Autodesk Fusion 360 part; units mm, degrees
(part 18 of 18)
  line L11330 (212.0954, -1.666) -> (212.0954, -1.906)
  line L11331 (211.6754, -1.666) -> (212.0954, -1.666)
  line L11332 (211.6754, -2.1661) -> (212.0954, -2.1661)
  line L11333 (212.0954, -2.1661) -> (212.0954, -2.4061)
  line L11334 (212.0954, -2.4061) -> (211.6754, -2.4061)
  line L11335 (211.6754, -2.4061) -> (211.6754, -2.1661)
  line L11336 (212.0954, -2.906) -> (211.6754, -2.906)
  line L11337 (211.6754, -2.666) -> (212.0954, -2.666)
  line L11338 (211.6754, -2.906) -> (211.6754, -2.666)
  line L11339 (212.0954, -2.666) -> (212.0954, -2.906)
  line L11340 (212.0954, -3.4059) -> (211.6754, -3.4059)
  line L11341 (211.6754, -3.1659) -> (212.0954, -3.1659)
  line L11342 (212.0954, -3.1659) -> (212.0954, -3.4059)
  line L11343 (211.6754, -3.4059) -> (211.6754, -3.1659)
  line L11344 (138.9953, -77.1606) -> (138.9953, -76.5606)
  line L11345 (138.7753, -77.1606) -> (138.9953, -77.1606)
  line L11346 (138.7753, -76.5606) -> (138.7753, -77.1606)
  line L11347 (138.9953, -76.5606) -> (138.7753, -76.5606)
  line L11348 (141.8953, -76.5606) -> (141.8953, -77.1606)
  line L11349 (141.6753, -77.1606) -> (141.6753, -76.5606)
  line L11350 (141.8953, -77.1606) -> (141.6753, -77.1606)
  line L11351 (141.6753, -76.5606) -> (141.8953, -76.5606)
  line L11352 (138.9953, -19.985) -> (138.9953, -19.385)
  line L11353 (138.7753, -19.385) -> (138.7753, -19.985)
  line L11354 (138.7753, -19.985) -> (138.9953, -19.985)
  line L11355 (138.9953, -19.385) -> (138.7753, -19.385)
  line L11356 (141.6753, -19.985) -> (141.6753, -19.385)
  line L11357 (141.8953, -19.985) -> (141.6753, -19.985)
  line L11358 (141.8953, -19.385) -> (141.8953, -19.985)
  line L11359 (141.6753, -19.385) -> (141.8953, -19.385)
  line L11360 (138.9953, -39.0351) -> (138.9953, -38.4351)
  line L11361 (138.7753, -39.0351) -> (138.9953, -39.0351)
  line L11362 (138.7753, -38.4351) -> (138.7753, -39.0351)
  line L11363 (138.9953, -38.4351) -> (138.7753, -38.4351)
  line L11364 (141.6753, -38.4351) -> (141.8953, -38.4351)
  line L11365 (141.6753, -39.0351) -> (141.6753, -38.4351)
  line L11366 (141.8953, -39.0351) -> (141.6753, -39.0351)
  line L11367 (141.8953, -38.4351) -> (141.8953, -39.0351)
  line L11368 (138.7753, -58.0978) -> (138.9953, -58.0978)
  line L11369 (138.9953, -58.0978) -> (138.9953, -57.4978)
  line L11370 (138.9953, -57.4978) -> (138.7753, -57.4978)
  line L11371 (138.7753, -57.4978) -> (138.7753, -58.0978)
  line L11372 (141.6753, -57.4978) -> (141.8953, -57.4978)
  line L11373 (141.8953, -57.4978) -> (141.8953, -58.0978)
  line L11374 (141.6753, -58.0978) -> (141.6753, -57.4978)
  line L11375 (141.8953, -58.0978) -> (141.6753, -58.0978)
  line L11376 (157.8253, -19.385) -> (157.8253, -19.985)
  line L11377 (157.8253, -19.985) -> (158.0453, -19.985)
  line L11378 (158.0453, -19.385) -> (157.8253, -19.385)
  line L11379 (158.0453, -19.985) -> (158.0453, -19.385)
  line L11380 (160.9453, -19.985) -> (160.7253, -19.985)
  line L11381 (160.7253, -19.985) -> (160.7253, -19.385)
  line L11382 (160.9453, -19.385) -> (160.9453, -19.985)
  line L11383 (160.7253, -19.385) -> (160.9453, -19.385)
  line L11384 (158.0453, -76.5606) -> (157.8253, -76.5606)
  line L11385 (157.8253, -77.1606) -> (158.0453, -77.1606)
  line L11386 (158.0453, -77.1606) -> (158.0453, -76.5606)
  line L11387 (157.8253, -76.5606) -> (157.8253, -77.1606)
  line L11388 (160.9453, -76.5606) -> (160.9453, -77.1606)
  line L11389 (160.9453, -77.1606) -> (160.7253, -77.1606)
  line L11390 (160.7253, -77.1606) -> (160.7253, -76.5606)
  line L11391 (160.7253, -76.5606) -> (160.9453, -76.5606)
  line L11392 (157.8253, -57.4978) -> (157.8253, -58.0978)
  line L11393 (157.8253, -58.0978) -> (158.0453, -58.0978)
  line L11394 (158.0453, -57.4978) -> (157.8253, -57.4978)
  line L11395 (158.0453, -58.0978) -> (158.0453, -57.4978)
  line L11396 (160.7253, -58.0978) -> (160.7253, -57.4978)
  line L11397 (160.9453, -58.0978) -> (160.7253, -58.0978)
  line L11398 (160.7253, -57.4978) -> (160.9453, -57.4978)
  line L11399 (160.9453, -57.4978) -> (160.9453, -58.0978)
  line L11400 (158.0453, -38.4351) -> (157.8253, -38.4351)
  line L11401 (157.8253, -38.4351) -> (157.8253, -39.0351)
  line L11402 (158.0453, -39.0351) -> (158.0453, -38.4351)
  line L11403 (157.8253, -39.0351) -> (158.0453, -39.0351)
  line L11404 (160.7253, -38.4351) -> (160.9453, -38.4351)
  line L11405 (160.7253, -39.0351) -> (160.7253, -38.4351)
  line L11406 (160.9453, -38.4351) -> (160.9453, -39.0351)
  line L11407 (160.9453, -39.0351) -> (160.7253, -39.0351)
  line L11408 (177.0954, -19.385) -> (176.8754, -19.385)
  line L11409 (176.8754, -19.385) -> (176.8754, -19.985)
  line L11410 (177.0954, -19.985) -> (177.0954, -19.385)
  line L11411 (176.8754, -19.985) -> (177.0954, -19.985)
  line L11412 (179.7754, -19.385) -> (179.9954, -19.385)
  line L11413 (179.7754, -19.985) -> (179.7754, -19.385)
  line L11414 (179.9954, -19.985) -> (179.7754, -19.985)
  line L11415 (179.9954, -19.385) -> (179.9954, -19.985)
  line L11416 (177.0954, -76.5606) -> (176.8754, -76.5606)
  line L11417 (176.8754, -77.1606) -> (177.0954, -77.1606)
  line L11418 (177.0954, -77.1606) -> (177.0954, -76.5606)
  line L11419 (176.8754, -76.5606) -> (176.8754, -77.1606)
  line L11420 (179.7754, -76.5606) -> (179.9954, -76.5606)
  line L11421 (179.9954, -77.1606) -> (179.7754, -77.1606)
  line L11422 (179.9954, -76.5606) -> (179.9954, -77.1606)
  line L11423 (179.7754, -77.1606) -> (179.7754, -76.5606)
  line L11424 (177.0954, -58.0978) -> (177.0954, -57.4978)
  line L11425 (176.8754, -57.4978) -> (176.8754, -58.0978)
  line L11426 (176.8754, -58.0978) -> (177.0954, -58.0978)
  line L11427 (177.0954, -57.4978) -> (176.8754, -57.4978)
  line L11428 (179.9954, -57.4978) -> (179.9954, -58.0978)
  line L11429 (179.9954, -58.0978) -> (179.7754, -58.0978)
  line L11430 (179.7754, -58.0978) -> (179.7754, -57.4978)
  line L11431 (179.7754, -57.4978) -> (179.9954, -57.4978)
  line L11432 (176.8754, -38.4351) -> (176.8754, -39.0351)
  line L11433 (177.0954, -38.4351) -> (176.8754, -38.4351)
  line L11434 (177.0954, -39.0351) -> (177.0954, -38.4351)
  line L11435 (176.8754, -39.0351) -> (177.0954, -39.0351)
  line L11436 (179.9954, -38.4351) -> (179.9954, -39.0351)
  line L11437 (179.7754, -39.0351) -> (179.7754, -38.4351)
  line L11438 (179.7754, -38.4351) -> (179.9954, -38.4351)
  line L11439 (179.9954, -39.0351) -> (179.7754, -39.0351)
  line L11440 (100.8952, -77.1606) -> (100.8952, -76.5606)
  line L11441 (100.6752, -76.5606) -> (100.6752, -77.1606)
  line L11442 (100.6752, -77.1606) -> (100.8952, -77.1606)
  line L11443 (100.8952, -76.5606) -> (100.6752, -76.5606)
  line L11444 (103.7952, -77.1606) -> (103.5752, -77.1606)
  line L11445 (103.7952, -76.5606) -> (103.7952, -77.1606)
  line L11446 (103.5752, -77.1606) -> (103.5752, -76.5606)
  line L11447 (103.5752, -76.5606) -> (103.7952, -76.5606)
  line L11448 (100.6752, -58.0978) -> (100.8952, -58.0978)
  line L11449 (100.8952, -57.4978) -> (100.6752, -57.4978)
  line L11450 (100.8952, -58.0978) -> (100.8952, -57.4978)
  line L11451 (100.6752, -57.4978) -> (100.6752, -58.0978)
  line L11452 (103.5752, -58.0978) -> (103.5752, -57.4978)
  line L11453 (103.7952, -57.4978) -> (103.7952, -58.0978)
  line L11454 (103.7952, -58.0978) -> (103.5752, -58.0978)
  line L11455 (103.5752, -57.4978) -> (103.7952, -57.4978)
  line L11456 (100.8952, -19.985) -> (100.8952, -19.385)
  line L11457 (100.8952, -19.385) -> (100.6752, -19.385)
  line L11458 (100.6752, -19.985) -> (100.8952, -19.985)
  line L11459 (100.6752, -19.385) -> (100.6752, -19.985)
  line L11460 (103.5752, -19.385) -> (103.7952, -19.385)
  line L11461 (103.7952, -19.985) -> (103.5752, -19.985)
  line L11462 (103.7952, -19.385) -> (103.7952, -19.985)
  line L11463 (103.5752, -19.985) -> (103.5752, -19.385)
  line L11464 (100.6752, -39.0351) -> (100.8952, -39.0351)
  line L11465 (100.8952, -39.0351) -> (100.8952, -38.4351)
  line L11466 (100.8952, -38.4351) -> (100.6752, -38.4351)
  line L11467 (100.6752, -38.4351) -> (100.6752, -39.0351)
  line L11468 (103.5752, -39.0351) -> (103.5752, -38.4351)
  line L11469 (103.5752, -38.4351) -> (103.7952, -38.4351)
  line L11470 (103.7952, -38.4351) -> (103.7952, -39.0351)
  line L11471 (103.7952, -39.0351) -> (103.5752, -39.0351)
  line L11472 (119.7252, -19.385) -> (119.7252, -19.985)
  line L11473 (119.9452, -19.985) -> (119.9452, -19.385)
  line L11474 (119.9452, -19.385) -> (119.7252, -19.385)
  line L11475 (119.7252, -19.985) -> (119.9452, -19.985)
  line L11476 (122.6252, -19.385) -> (122.8452, -19.385)
  line L11477 (122.6252, -19.985) -> (122.6252, -19.385)
  line L11478 (122.8452, -19.385) -> (122.8452, -19.985)
  line L11479 (122.8452, -19.985) -> (122.6252, -19.985)
  line L11480 (119.7252, -57.4978) -> (119.7252, -58.0978)
  line L11481 (119.9452, -57.4978) -> (119.7252, -57.4978)
  line L11482 (119.9452, -58.0978) -> (119.9452, -57.4978)
  line L11483 (119.7252, -58.0978) -> (119.9452, -58.0978)
  line L11484 (122.6252, -57.4978) -> (122.8452, -57.4978)
  line L11485 (122.6252, -58.0978) -> (122.6252, -57.4978)
  line L11486 (122.8452, -57.4978) -> (122.8452, -58.0978)
  line L11487 (122.8452, -58.0978) -> (122.6252, -58.0978)
  line L11488 (119.9452, -39.0351) -> (119.9452, -38.4351)
  line L11489 (119.9452, -38.4351) -> (119.7252, -38.4351)
  line L11490 (119.7252, -38.4351) -> (119.7252, -39.0351)
  line L11491 (119.7252, -39.0351) -> (119.9452, -39.0351)
  line L11492 (122.8452, -38.4351) -> (122.8452, -39.0351)
  line L11493 (122.8452, -39.0351) -> (122.6252, -39.0351)
  line L11494 (122.6252, -38.4351) -> (122.8452, -38.4351)
  line L11495 (122.6252, -39.0351) -> (122.6252, -38.4351)
  line L11496 (119.9452, -76.5606) -> (119.7252, -76.5606)
  line L11497 (119.9452, -77.1606) -> (119.9452, -76.5606)
  line L11498 (119.7252, -77.1606) -> (119.9452, -77.1606)
  line L11499 (119.7252, -76.5606) -> (119.7252, -77.1606)
  line L11500 (122.6252, -76.5606) -> (122.8452, -76.5606)
  line L11501 (122.6252, -77.1606) -> (122.6252, -76.5606)
  line L11502 (122.8452, -76.5606) -> (122.8452, -77.1606)
  line L11503 (122.8452, -77.1606) -> (122.6252, -77.1606)
  line L11504 (5.425, -76.5606) -> (5.425, -77.1606)
  line L11505 (5.425, -77.1606) -> (5.645, -77.1606)
  line L11506 (5.645, -76.5606) -> (5.425, -76.5606)
  line L11507 (5.645, -77.1606) -> (5.645, -76.5606)
  line L11508 (8.545, -76.5606) -> (8.545, -77.1606)
  line L11509 (8.325, -77.1606) -> (8.325, -76.5606)
  line L11510 (8.545, -77.1606) -> (8.325, -77.1606)
  line L11511 (8.325, -76.5606) -> (8.545, -76.5606)
  line L11512 (24.4751, -77.1606) -> (24.6951, -77.1606)
  line L11513 (24.4751, -76.5606) -> (24.4751, -77.1606)
  line L11514 (24.6951, -77.1606) -> (24.6951, -76.5606)
  line L11515 (24.6951, -76.5606) -> (24.4751, -76.5606)
  line L11516 (27.5951, -77.1606) -> (27.3751, -77.1606)
  line L11517 (27.3751, -76.5606) -> (27.5951, -76.5606)
  line L11518 (27.3751, -77.1606) -> (27.3751, -76.5606)
  line L11519 (27.5951, -76.5606) -> (27.5951, -77.1606)
  line L11520 (43.7451, -76.5606) -> (43.5251, -76.5606)
  line L11521 (43.5251, -76.5606) -> (43.5251, -77.1606)
  line L11522 (43.5251, -77.1606) -> (43.7451, -77.1606)
  line L11523 (43.7451, -77.1606) -> (43.7451, -76.5606)
  line L11524 (46.6451, -77.1606) -> (46.4251, -77.1606)
  line L11525 (46.6451, -76.5606) -> (46.6451, -77.1606)
  line L11526 (46.4251, -77.1606) -> (46.4251, -76.5606)
  line L11527 (46.4251, -76.5606) -> (46.6451, -76.5606)
  line L11528 (62.5751, -19.985) -> (62.7951, -19.985)
  line L11529 (62.5751, -19.385) -> (62.5751, -19.985)
  line L11530 (62.7951, -19.385) -> (62.5751, -19.385)
  line L11531 (62.7951, -19.985) -> (62.7951, -19.385)
  line L11532 (65.6951, -19.985) -> (65.4751, -19.985)
  line L11533 (65.4751, -19.985) -> (65.4751, -19.385)
  line L11534 (65.6951, -19.385) -> (65.6951, -19.985)
  line L11535 (65.4751, -19.385) -> (65.6951, -19.385)
  line L11536 (62.5751, -77.1606) -> (62.7951, -77.1606)
  line L11537 (62.5751, -76.5606) -> (62.5751, -77.1606)
  line L11538 (62.7951, -76.5606) -> (62.5751, -76.5606)
  line L11539 (62.7951, -77.1606) -> (62.7951, -76.5606)
  line L11540 (65.6951, -77.1606) -> (65.4751, -77.1606)
  line L11541 (65.6951, -76.5606) -> (65.6951, -77.1606)
  line L11542 (65.4751, -77.1606) -> (65.4751, -76.5606)
  line L11543 (65.4751, -76.5606) -> (65.6951, -76.5606)
  line L11544 (62.7951, -39.0351) -> (62.7951, -38.4351)
  line L11545 (62.7951, -38.4351) -> (62.5751, -38.4351)
  line L11546 (62.5751, -39.0351) -> (62.7951, -39.0351)
  line L11547 (62.5751, -38.4351) -> (62.5751, -39.0351)
  line L11548 (65.6951, -39.0351) -> (65.4751, -39.0351)
  line L11549 (65.6951, -38.4351) -> (65.6951, -39.0351)
  line L11550 (65.4751, -39.0351) -> (65.4751, -38.4351)
  line L11551 (65.4751, -38.4351) -> (65.6951, -38.4351)
  line L11552 (62.7951, -57.4978) -> (62.5751, -57.4978)
  line L11553 (62.7951, -58.0978) -> (62.7951, -57.4978)
  line L11554 (62.5751, -57.4978) -> (62.5751, -58.0978)
  line L11555 (62.5751, -58.0978) -> (62.7951, -58.0978)
  line L11556 (65.4751, -57.4978) -> (65.6951, -57.4978)
  line L11557 (65.6951, -57.4978) -> (65.6951, -58.0978)
  line L11558 (65.6951, -58.0978) -> (65.4751, -58.0978)
  line L11559 (65.4751, -58.0978) -> (65.4751, -57.4978)
  line L11560 (81.8452, -39.0351) -> (81.8452, -38.4351)
  line L11561 (81.6252, -38.4351) -> (81.6252, -39.0351)
  line L11562 (81.8452, -38.4351) -> (81.6252, -38.4351)
  line L11563 (81.6252, -39.0351) -> (81.8452, -39.0351)
  line L11564 (84.5252, -39.0351) -> (84.5252, -38.4351)
  line L11565 (84.7452, -38.4351) -> (84.7452, -39.0351)
  line L11566 (84.7452, -39.0351) -> (84.5252, -39.0351)
  line L11567 (84.5252, -38.4351) -> (84.7452, -38.4351)
  line L11568 (81.6252, -76.5606) -> (81.6252, -77.1606)
  line L11569 (81.6252, -77.1606) -> (81.8452, -77.1606)
  line L11570 (81.8452, -77.1606) -> (81.8452, -76.5606)
  line L11571 (81.8452, -76.5606) -> (81.6252, -76.5606)
  line L11572 (84.7452, -76.5606) -> (84.7452, -77.1606)
  line L11573 (84.7452, -77.1606) -> (84.5252, -77.1606)
  line L11574 (84.5252, -77.1606) -> (84.5252, -76.5606)
  line L11575 (84.5252, -76.5606) -> (84.7452, -76.5606)
  line L11576 (81.6252, -19.385) -> (81.6252, -19.985)
  line L11577 (81.8452, -19.985) -> (81.8452, -19.385)
  line L11578 (81.8452, -19.385) -> (81.6252, -19.385)
  line L11579 (81.6252, -19.985) -> (81.8452, -19.985)
  line L11580 (84.7452, -19.385) -> (84.7452, -19.985)
  line L11581 (84.7452, -19.985) -> (84.5252, -19.985)
  line L11582 (84.5252, -19.985) -> (84.5252, -19.385)
  line L11583 (84.5252, -19.385) -> (84.7452, -19.385)
  line L11584 (81.8452, -58.0978) -> (81.8452, -57.4978)
  line L11585 (81.6252, -57.4978) -> (81.6252, -58.0978)
  line L11586 (81.8452, -57.4978) -> (81.6252, -57.4978)
  line L11587 (81.6252, -58.0978) -> (81.8452, -58.0978)
  line L11588 (84.7452, -58.0978) -> (84.5252, -58.0978)
  line L11589 (84.7452, -57.4978) -> (84.7452, -58.0978)
  line L11590 (84.5252, -57.4978) -> (84.7452, -57.4978)
  line L11591 (84.5252, -58.0978) -> (84.5252, -57.4978)
  line L11592 (5.425, -57.4978) -> (5.425, -58.0978)
  line L11593 (5.645, -58.0978) -> (5.645, -57.4978)
  line L11594 (5.425, -58.0978) -> (5.645, -58.0978)
  line L11595 (5.645, -57.4978) -> (5.425, -57.4978)
  line L11596 (8.545, -57.4978) -> (8.545, -58.0978)
  line L11597 (8.545, -58.0978) -> (8.325, -58.0978)
  line L11598 (8.325, -57.4978) -> (8.545, -57.4978)
  line L11599 (8.325, -58.0978) -> (8.325, -57.4978)
  line L11600 (5.425, -19.985) -> (5.645, -19.985)
  line L11601 (5.425, -19.385) -> (5.425, -19.985)
  line L11602 (5.645, -19.385) -> (5.425, -19.385)
  line L11603 (5.645, -19.985) -> (5.645, -19.385)
  line L11604 (8.325, -19.985) -> (8.325, -19.385)
  line L11605 (8.545, -19.385) -> (8.545, -19.985)
  line L11606 (8.545, -19.985) -> (8.325, -19.985)
  line L11607 (8.325, -19.385) -> (8.545, -19.385)
  line L11608 (5.425, -38.4351) -> (5.425, -39.0351)
  line L11609 (5.425, -39.0351) -> (5.645, -39.0351)
  line L11610 (5.645, -39.0351) -> (5.645, -38.4351)
  line L11611 (5.645, -38.4351) -> (5.425, -38.4351)
  line L11612 (8.325, -38.4351) -> (8.545, -38.4351)
  line L11613 (8.325, -39.0351) -> (8.325, -38.4351)
  line L11614 (8.545, -38.4351) -> (8.545, -39.0351)
  line L11615 (8.545, -39.0351) -> (8.325, -39.0351)
  line L11616 (24.6951, -38.4351) -> (24.4751, -38.4351)
  line L11617 (24.4751, -38.4351) -> (24.4751, -39.0351)
  line L11618 (24.4751, -39.0351) -> (24.6951, -39.0351)
  line L11619 (24.6951, -39.0351) -> (24.6951, -38.4351)
  line L11620 (27.5951, -38.4351) -> (27.5951, -39.0351)
  line L11621 (27.3751, -38.4351) -> (27.5951, -38.4351)
  line L11622 (27.3751, -39.0351) -> (27.3751, -38.4351)
  line L11623 (27.5951, -39.0351) -> (27.3751, -39.0351)
  line L11624 (24.6951, -19.985) -> (24.6951, -19.385)
  line L11625 (24.6951, -19.385) -> (24.4751, -19.385)
  line L11626 (24.4751, -19.385) -> (24.4751, -19.985)
  line L11627 (24.4751, -19.985) -> (24.6951, -19.985)
  line L11628 (27.5951, -19.985) -> (27.3751, -19.985)
  line L11629 (27.5951, -19.385) -> (27.5951, -19.985)
  line L11630 (27.3751, -19.385) -> (27.5951, -19.385)
  line L11631 (27.3751, -19.985) -> (27.3751, -19.385)
  line L11632 (24.6951, -57.4978) -> (24.4751, -57.4978)
  line L11633 (24.4751, -58.0978) -> (24.6951, -58.0978)
  line L11634 (24.4751, -57.4978) -> (24.4751, -58.0978)
  line L11635 (24.6951, -58.0978) -> (24.6951, -57.4978)
  line L11636 (27.5951, -58.0978) -> (27.3751, -58.0978)
  line L11637 (27.5951, -57.4978) -> (27.5951, -58.0978)
  line L11638 (27.3751, -57.4978) -> (27.5951, -57.4978)
  line L11639 (27.3751, -58.0978) -> (27.3751, -57.4978)
  line L11640 (43.7451, -19.385) -> (43.5251, -19.385)
  line L11641 (43.7451, -19.985) -> (43.7451, -19.385)
  line L11642 (43.5251, -19.985) -> (43.7451, -19.985)
  line L11643 (43.5251, -19.385) -> (43.5251, -19.985)
  line L11644 (46.4251, -19.385) -> (46.6451, -19.385)
  line L11645 (46.6451, -19.985) -> (46.4251, -19.985)
  line L11646 (46.6451, -19.385) -> (46.6451, -19.985)
  line L11647 (46.4251, -19.985) -> (46.4251, -19.385)
  line L11648 (43.5251, -57.4978) -> (43.5251, -58.0978)
  line L11649 (43.5251, -58.0978) -> (43.7451, -58.0978)
  line L11650 (43.7451, -58.0978) -> (43.7451, -57.4978)
  line L11651 (43.7451, -57.4978) -> (43.5251, -57.4978)
  line L11652 (46.4251, -58.0978) -> (46.4251, -57.4978)
  line L11653 (46.4251, -57.4978) -> (46.6451, -57.4978)
  line L11654 (46.6451, -57.4978) -> (46.6451, -58.0978)
  line L11655 (46.6451, -58.0978) -> (46.4251, -58.0978)
  line L11656 (43.5251, -39.0351) -> (43.7451, -39.0351)
  line L11657 (43.5251, -38.4351) -> (43.5251, -39.0351)
  line L11658 (43.7451, -38.4351) -> (43.5251, -38.4351)
  line L11659 (43.7451, -39.0351) -> (43.7451, -38.4351)
  line L11660 (46.6451, -38.4351) -> (46.6451, -39.0351)
  line L11661 (46.6451, -39.0351) -> (46.4251, -39.0351)
  line L11662 (46.4251, -38.4351) -> (46.6451, -38.4351)
  line L11663 (46.4251, -39.0351) -> (46.4251, -38.4351)
  line L11664 (215.1954, -19.385) -> (214.9754, -19.385)
  line L11665 (214.9754, -19.385) -> (214.9754, -19.985)
  line L11666 (215.1954, -19.985) -> (215.1954, -19.385)
  line L11667 (214.9754, -19.985) -> (215.1954, -19.985)
  line L11668 (217.8754, -19.385) -> (218.0954, -19.385)
  line L11669 (218.0954, -19.985) -> (217.8754, -19.985)
  line L11670 (217.8754, -19.985) -> (217.8754, -19.385)
  line L11671 (218.0954, -19.385) -> (218.0954, -19.985)
  line L11672 (215.1954, -76.5606) -> (214.9754, -76.5606)
  line L11673 (214.9754, -76.5606) -> (214.9754, -77.1606)
  line L11674 (215.1954, -77.1606) -> (215.1954, -76.5606)
  line L11675 (214.9754, -77.1606) -> (215.1954, -77.1606)
  line L11676 (217.8754, -77.1606) -> (217.8754, -76.5606)
  line L11677 (218.0954, -77.1606) -> (217.8754, -77.1606)
  line L11678 (217.8754, -76.5606) -> (218.0954, -76.5606)
  line L11679 (218.0954, -76.5606) -> (218.0954, -77.1606)
  line L11680 (215.1954, -57.4978) -> (214.9754, -57.4978)
  line L11681 (214.9754, -57.4978) -> (214.9754, -58.0978)
  line L11682 (215.1954, -58.0978) -> (215.1954, -57.4978)
  line L11683 (214.9754, -58.0978) -> (215.1954, -58.0978)
  line L11684 (217.8754, -58.0978) -> (217.8754, -57.4978)
  line L11685 (217.8754, -57.4978) -> (218.0954, -57.4978)
  line L11686 (218.0954, -58.0978) -> (217.8754, -58.0978)
  line L11687 (218.0954, -57.4978) -> (218.0954, -58.0978)
  line L11688 (215.1954, -38.4351) -> (214.9754, -38.4351)
  line L11689 (214.9754, -38.4351) -> (214.9754, -39.0351)
  line L11690 (214.9754, -39.0351) -> (215.1954, -39.0351)
  line L11691 (215.1954, -39.0351) -> (215.1954, -38.4351)
  line L11692 (217.8754, -38.4351) -> (218.0954, -38.4351)
  line L11693 (218.0954, -39.0351) -> (217.8754, -39.0351)
  line L11694 (218.0954, -38.4351) -> (218.0954, -39.0351)
  line L11695 (217.8754, -39.0351) -> (217.8754, -38.4351)
  line L11696 (196.1454, -38.4351) -> (195.9254, -38.4351)
  line L11697 (195.9254, -38.4351) -> (195.9254, -39.0351)
  line L11698 (195.9254, -39.0351) -> (196.1454, -39.0351)
  line L11699 (196.1454, -39.0351) -> (196.1454, -38.4351)
  line L11700 (199.0454, -39.0351) -> (198.8254, -39.0351)
  line L11701 (198.8254, -39.0351) -> (198.8254, -38.4351)
  line L11702 (199.0454, -38.4351) -> (199.0454, -39.0351)
  line L11703 (198.8254, -38.4351) -> (199.0454, -38.4351)
  line L11704 (195.9254, -77.1606) -> (196.1454, -77.1606)
  line L11705 (196.1454, -77.1606) -> (196.1454, -76.5606)
  line L11706 (196.1454, -76.5606) -> (195.9254, -76.5606)
  line L11707 (195.9254, -76.5606) -> (195.9254, -77.1606)
  line L11708 (199.0454, -77.1606) -> (198.8254, -77.1606)
  line L11709 (198.8254, -76.5606) -> (199.0454, -76.5606)
  line L11710 (199.0454, -76.5606) -> (199.0454, -77.1606)
  line L11711 (198.8254, -77.1606) -> (198.8254, -76.5606)
  line L11712 (196.1454, -57.4978) -> (195.9254, -57.4978)
  line L11713 (195.9254, -57.4978) -> (195.9254, -58.0978)
  line L11714 (196.1454, -58.0978) -> (196.1454, -57.4978)
  line L11715 (195.9254, -58.0978) -> (196.1454, -58.0978)
  line L11716 (199.0454, -58.0978) -> (198.8254, -58.0978)
  line L11717 (198.8254, -58.0978) -> (198.8254, -57.4978)
  line L11718 (199.0454, -57.4978) -> (199.0454, -58.0978)
  line L11719 (198.8254, -57.4978) -> (199.0454, -57.4978)
  line L11720 (196.1454, -19.385) -> (195.9254, -19.385)
  line L11721 (195.9254, -19.385) -> (195.9254, -19.985)
  line L11722 (195.9254, -19.985) -> (196.1454, -19.985)
  line L11723 (196.1454, -19.985) -> (196.1454, -19.385)
  line L11724 (198.8254, -19.985) -> (198.8254, -19.385)
  line L11725 (199.0454, -19.985) -> (198.8254, -19.985)
  line L11726 (199.0454, -19.385) -> (199.0454, -19.985)
  line L11727 (198.8254, -19.385) -> (199.0454, -19.385)
  line L11728 (197.1272, -3.67) -> (197.1272, -3.92)
  line L11729 (197.1272, -3.92) -> (196.9422, -3.92)
  line L11730 (196.9422, -3.67) -> (197.1272, -3.67)
  line L11731 (196.9422, -3.92) -> (196.9422, -3.67)
  line L11732 (196.9421, -4.97) -> (197.1271, -4.97)
  line L11733 (197.1271, -5.22) -> (196.9421, -5.22)
  line L11734 (196.9421, -5.22) -> (196.9421, -4.97)
  line L11735 (197.1271, -4.97) -> (197.1271, -5.22)
  line L11736 (195.7274, -3.67) -> (195.7274, -3.92)
  line L11737 (195.5424, -3.92) -> (195.5424, -3.67)
  line L11738 (195.7274, -3.92) -> (195.5424, -3.92)
  line L11739 (195.5424, -3.67) -> (195.7274, -3.67)
  line L11740 (195.7274, -4.32) -> (195.7274, -4.57)
  line L11741 (195.5424, -4.57) -> (195.5424, -4.32)
  line L11742 (195.5424, -4.32) -> (195.7274, -4.32)
  line L11743 (195.7274, -4.57) -> (195.5424, -4.57)
  line L11744 (195.5424, -5.22) -> (195.5424, -4.97)
  line L11745 (195.7274, -4.97) -> (195.7274, -5.22)
  line L11746 (195.5424, -4.97) -> (195.7274, -4.97)
  line L11747 (195.7274, -5.22) -> (195.5424, -5.22)
sketch "草图3" plane through (0, 0, 0) normal (0, 0, 1) x (1, 0, 0)
  line L0 (-5.6, -12.4) -> (8.45, -12.4)
  line L1 (8.45, -12.4) -> (8.45, -26.45)
  line L2 (8.45, -26.45) -> (-5.6, -26.45)
  line L3 (-5.6, -26.45) -> (-5.6, -12.4)
  line L4 (13.45, -26.45) -> (13.45, -12.4)
  line L5 (13.45, -12.4) -> (27.5, -12.4)
  line L6 (27.5, -12.4) -> (27.5, -26.45)
  line L7 (27.5, -26.45) -> (13.45, -26.45)
  line L8 (32.5, -26.45) -> (32.5, -12.4)
  line L9 (32.5, -12.4) -> (46.55, -12.4)
  line L10 (46.55, -12.4) -> (46.55, -26.45)
  line L11 (46.55, -26.45) -> (32.5, -26.45)
  line L12 (51.55, -26.45) -> (51.55, -12.4)
  line L13 (51.55, -12.4) -> (65.6, -12.4)
  line L14 (65.6, -12.4) -> (65.6, -26.45)
  line L15 (65.6, -26.45) -> (51.55, -26.45)
  line L16 (70.6, -26.45) -> (70.6, -12.4)
  line L17 (70.6, -12.4) -> (84.65, -12.4)
  line L18 (84.65, -12.4) -> (84.65, -26.45)
  line L19 (84.65, -26.45) -> (70.6, -26.45)
  line L20 (89.65, -26.45) -> (89.65, -12.4)
  line L21 (89.65, -12.4) -> (103.7, -12.4)
  line L22 (103.7, -12.4) -> (103.7, -26.45)
  line L23 (103.7, -26.45) -> (89.65, -26.45)
  line L24 (108.7, -26.45) -> (108.7, -12.4)
  line L25 (108.7, -12.4) -> (122.75, -12.4)
  line L26 (122.75, -12.4) -> (122.75, -26.45)
  line L27 (122.75, -26.45) -> (108.7, -26.45)
  line L28 (127.75, -26.45) -> (127.75, -12.4)
  line L29 (127.75, -12.4) -> (141.8, -12.4)
  line L30 (141.8, -12.4) -> (141.8, -26.45)
  line L31 (141.8, -26.45) -> (127.75, -26.45)
  line L32 (146.8, -26.45) -> (146.8, -12.4)
  line L33 (146.8, -12.4) -> (160.85, -12.4)
  line L34 (160.85, -12.4) -> (160.85, -26.45)
  line L35 (160.85, -26.45) -> (146.8, -26.45)
  line L36 (165.85, -26.45) -> (165.85, -12.4)
  line L37 (165.85, -12.4) -> (179.9, -12.4)
  line L38 (179.9, -12.4) -> (179.9, -26.45)
  line L39 (179.9, -26.45) -> (165.85, -26.45)
  line L40 (184.9, -26.45) -> (184.9, -12.4)
  line L41 (184.9, -12.4) -> (198.95, -12.4)
  line L42 (198.95, -12.4) -> (198.95, -26.45)
  line L43 (198.95, -26.45) -> (184.9, -26.45)
  line L44 (203.95, -26.45) -> (203.95, -12.4)
  line L45 (203.95, -12.4) -> (218, -12.4)
  line L46 (218, -12.4) -> (218, -26.45)
  line L47 (218, -26.45) -> (203.95, -26.45)
  line L48 (-5.6, -45.5) -> (-5.6, -31.45)
  line L49 (-5.6, -31.45) -> (8.45, -31.45)
  line L50 (8.45, -31.45) -> (8.45, -45.5)
  line L51 (8.45, -45.5) -> (-5.6, -45.5)
  line L52 (13.45, -45.5) -> (13.45, -31.45)
  line L53 (13.45, -31.45) -> (27.5, -31.45)
  line L54 (27.5, -31.45) -> (27.5, -45.5)
  line L55 (27.5, -45.5) -> (13.45, -45.5)
  line L56 (32.5, -45.5) -> (32.5, -31.45)
  line L57 (32.5, -31.45) -> (46.55, -31.45)
  line L58 (46.55, -31.45) -> (46.55, -45.5)
  line L59 (46.55, -45.5) -> (32.5, -45.5)
  line L60 (51.55, -45.5) -> (51.55, -31.45)
  line L61 (51.55, -31.45) -> (65.6, -31.45)
  line L62 (65.6, -31.45) -> (65.6, -45.5)
  line L63 (65.6, -45.5) -> (51.55, -45.5)
  line L64 (70.6, -45.5) -> (70.6, -31.45)
  line L65 (70.6, -31.45) -> (84.65, -31.45)
  line L66 (84.65, -31.45) -> (84.65, -45.5)
  line L67 (84.65, -45.5) -> (70.6, -45.5)
  line L68 (89.65, -45.5) -> (89.65, -31.45)
  line L69 (89.65, -31.45) -> (103.7, -31.45)
  line L70 (103.7, -31.45) -> (103.7, -45.5)
  line L71 (103.7, -45.5) -> (89.65, -45.5)
  line L72 (108.7, -45.5) -> (108.7, -31.45)
  line L73 (108.7, -31.45) -> (122.75, -31.45)
  line L74 (122.75, -31.45) -> (122.75, -45.5)
  line L75 (122.75, -45.5) -> (108.7, -45.5)
  line L76 (127.75, -45.5) -> (127.75, -31.45)
  line L77 (127.75, -31.45) -> (141.8, -31.45)
  line L78 (141.8, -31.45) -> (141.8, -45.5)
  line L79 (141.8, -45.5) -> (127.75, -45.5)
  line L80 (146.8, -45.5) -> (146.8, -31.45)
  line L81 (146.8, -31.45) -> (160.85, -31.45)
  line L82 (160.85, -31.45) -> (160.85, -45.5)
  line L83 (160.85, -45.5) -> (146.8, -45.5)
  line L84 (165.85, -45.5) -> (165.85, -31.45)
  line L85 (165.85, -31.45) -> (179.9, -31.45)
  line L86 (179.9, -31.45) -> (179.9, -45.5)
  line L87 (179.9, -45.5) -> (165.85, -45.5)
  line L88 (184.9, -45.5) -> (184.9, -31.45)
  line L89 (184.9, -31.45) -> (198.95, -31.45)
  line L90 (198.95, -31.45) -> (198.95, -45.5)
  line L91 (198.95, -45.5) -> (184.9, -45.5)
  line L92 (203.95, -45.5) -> (203.95, -31.45)
  line L93 (203.95, -31.45) -> (218, -31.45)
  line L94 (218, -31.45) -> (218, -45.5)
  line L95 (218, -45.5) -> (203.95, -45.5)
  line L96 (-5.6, -64.55) -> (-5.6, -50.5)
  line L97 (-5.6, -50.5) -> (8.45, -50.5)
  line L98 (8.45, -50.5) -> (8.45, -64.55)
  line L99 (8.45, -64.55) -> (-5.6, -64.55)
  line L100 (13.45, -64.55) -> (13.45, -50.5)
  line L101 (13.45, -50.5) -> (27.5, -50.5)
  line L102 (27.5, -50.5) -> (27.5, -64.55)
  line L103 (27.5, -64.55) -> (13.45, -64.55)
  line L104 (32.5, -64.55) -> (32.5, -50.5)
  line L105 (32.5, -50.5) -> (46.55, -50.5)
  line L106 (46.55, -50.5) -> (46.55, -64.55)
  line L107 (46.55, -64.55) -> (32.5, -64.55)
  line L108 (51.55, -64.55) -> (51.55, -50.5)
  line L109 (51.55, -50.5) -> (65.6, -50.5)
  line L110 (65.6, -50.5) -> (65.6, -64.55)
  line L111 (65.6, -64.55) -> (51.55, -64.55)
  line L112 (70.6, -64.55) -> (70.6, -50.5)
  line L113 (70.6, -50.5) -> (84.65, -50.5)
  line L114 (84.65, -50.5) -> (84.65, -64.55)
  line L115 (84.65, -64.55) -> (70.6, -64.55)
  line L116 (89.65, -64.55) -> (89.65, -50.5)
  line L117 (89.65, -50.5) -> (103.7, -50.5)
  line L118 (103.7, -50.5) -> (103.7, -64.55)
  line L119 (103.7, -64.55) -> (89.65, -64.55)
  line L120 (108.7, -64.55) -> (108.7, -50.5)
  line L121 (108.7, -50.5) -> (122.75, -50.5)
  line L122 (122.75, -50.5) -> (122.75, -64.55)
  line L123 (122.75, -64.55) -> (108.7, -64.55)
  line L124 (127.75, -64.55) -> (127.75, -50.5)
  line L125 (127.75, -50.5) -> (141.8, -50.5)
  line L126 (141.8, -50.5) -> (141.8, -64.55)
  line L127 (141.8, -64.55) -> (127.75, -64.55)
  line L128 (146.8, -64.55) -> (146.8, -50.5)
  line L129 (146.8, -50.5) -> (160.85, -50.5)
  line L130 (160.85, -50.5) -> (160.85, -64.55)
  line L131 (160.85, -64.55) -> (146.8, -64.55)
  line L132 (165.85, -64.55) -> (165.85, -50.5)
  line L133 (165.85, -50.5) -> (179.9, -50.5)
  line L134 (179.9, -50.5) -> (179.9, -64.55)
  line L135 (179.9, -64.55) -> (165.85, -64.55)
  line L136 (184.9, -64.55) -> (184.9, -50.5)
  line L137 (184.9, -50.5) -> (198.95, -50.5)
  line L138 (198.95, -50.5) -> (198.95, -64.55)
  line L139 (198.95, -64.55) -> (184.9, -64.55)
  line L140 (203.95, -64.55) -> (203.95, -50.5)
  line L141 (203.95, -50.5) -> (218, -50.5)
  line L142 (218, -50.5) -> (218, -64.55)
  line L143 (218, -64.55) -> (203.95, -64.55)
  line L144 (-5.6, -83.6) -> (-5.6, -69.55)
  line L145 (-5.6, -69.55) -> (8.45, -69.55)
  line L146 (8.45, -69.55) -> (8.45, -83.6)
  line L147 (8.45, -83.6) -> (-5.6, -83.6)
  line L148 (13.45, -83.6) -> (13.45, -69.55)
  line L149 (13.45, -69.55) -> (27.5, -69.55)
  line L150 (27.5, -69.55) -> (27.5, -83.6)
  line L151 (27.5, -83.6) -> (13.45, -83.6)
  line L152 (32.5, -83.6) -> (32.5, -69.55)
  line L153 (32.5, -69.55) -> (46.55, -69.55)
  line L154 (46.55, -69.55) -> (46.55, -83.6)
  line L155 (46.55, -83.6) -> (32.5, -83.6)
  line L156 (51.55, -83.6) -> (51.55, -69.55)
  line L157 (51.55, -69.55) -> (65.6, -69.55)
  line L158 (65.6, -69.55) -> (65.6, -83.6)
  line L159 (65.6, -83.6) -> (51.55, -83.6)
  line L160 (70.6, -83.6) -> (70.6, -69.55)
  line L161 (70.6, -69.55) -> (84.65, -69.55)
  line L162 (84.65, -69.55) -> (84.65, -83.6)
  line L163 (84.65, -83.6) -> (70.6, -83.6)
  line L164 (89.65, -83.6) -> (89.65, -69.55)
  line L165 (89.65, -69.55) -> (103.7, -69.55)
  line L166 (103.7, -69.55) -> (103.7, -83.6)
  line L167 (103.7, -83.6) -> (89.65, -83.6)
  line L168 (108.7, -83.6) -> (108.7, -69.55)
  line L169 (108.7, -69.55) -> (122.75, -69.55)
  line L170 (122.75, -69.55) -> (122.75, -83.6)
  line L171 (122.75, -83.6) -> (108.7, -83.6)
  line L172 (127.75, -83.6) -> (127.75, -69.55)
  line L173 (127.75, -69.55) -> (141.8, -69.55)
  line L174 (141.8, -69.55) -> (141.8, -83.6)
  line L175 (141.8, -83.6) -> (127.75, -83.6)
  line L176 (146.8, -83.6) -> (146.8, -69.55)
  line L177 (146.8, -69.55) -> (160.85, -69.55)
  line L178 (160.85, -69.55) -> (160.85, -83.6)
  line L179 (160.85, -83.6) -> (146.8, -83.6)
  line L180 (165.85, -83.6) -> (165.85, -69.55)
  line L181 (165.85, -69.55) -> (179.9, -69.55)
  line L182 (179.9, -69.55) -> (179.9, -83.6)
  line L183 (179.9, -83.6) -> (165.85, -83.6)
  line L184 (184.9, -83.6) -> (184.9, -69.55)
  line L185 (184.9, -69.55) -> (198.95, -69.55)
  line L186 (198.95, -69.55) -> (198.95, -83.6)
  line L187 (198.95, -83.6) -> (184.9, -83.6)
  line L188 (203.95, -83.6) -> (203.95, -69.55)
  line L189 (203.95, -69.55) -> (218, -69.55)
  line L190 (218, -69.55) -> (218, -83.6)
  line L191 (218, -83.6) -> (203.95, -83.6)
  circle A0 centre (2.1385, -5.4604) radius 3.3897
  dimension "d1" = 14.05
  dimension "d2" = 14.05
  dimension "d5" = 19.05
  dimension "d6" = -19.05
  constraint horizontal L0
  constraint vertical L1
  constraint horizontal L2
  constraint vertical L3
  measures "d1" distance of L0.start L0.end
  measures "d2" distance of L0.start L2.end
sketch "草图4" plane through (0, 0, 0) normal (0, 0, 1) x (1, 0, 0)
  line L0 (-10.6937, 1.6265) -> (222.987, 1.6265)
  line L1 (222.987, 1.6265) -> (222.987, -88.5449)
  line L2 (222.987, -88.5449) -> (-10.6937, -88.5449)
  line L3 (-10.6937, -88.5449) -> (-10.6937, 1.6265)
  line L4 (-13.6937, 4.6265) -> (225.987, 4.6265)
  line L5 (225.987, 4.6265) -> (225.987, -91.5449)
  line L6 (225.987, -91.5449) -> (-13.6937, -91.5449)
  line L7 (-13.6937, -91.5449) -> (-13.6937, 4.6265)
  dimension "d11" = -3
  constraint horizontal L0
  constraint vertical L1
  constraint horizontal L2
  constraint vertical L3
extrude "拉伸3" add sketch "草图4" against normal blind 8.5 makes body 1
extrude "拉伸4" add 1 faces at (67.1999, -90.5449, -8.5) along direction (0, 0, -1) blind 2.5 separate body on bodies 1 makes body 2
sketch "草图5" plane through (0, 0, 0) normal (0, 0, 1) x (1, 0, 0)
  line L0 (-13.6937, -91.5449) -> (225.9869, -91.5449)
  line L1 (225.9869, -91.5449) -> (225.9869, 4.6266)
  line L2 (225.9869, 4.6266) -> (-13.6937, 4.6266)
  line L3 (-13.6937, 4.6266) -> (-13.6937, -91.5449)
  constraint horizontal L0
  constraint vertical L1
  constraint horizontal L2
  constraint vertical L3
sketch "草图7" plane through (0, 0, -11) normal (0, 0, -1) x (1, 0, 0)
  line L0 (-10.6937, 88.5449) -> (222.987, 88.5449)
  line L1 (222.987, 88.5449) -> (222.987, -1.6265)
  line L2 (222.987, -1.6265) -> (-10.6937, -1.6265)
  line L3 (-10.6937, -1.6265) -> (-10.6937, 88.5449)
  line L4 (225.987, 91.5449) -> (-13.6937, 91.5449)
  line L5 (-13.6937, 91.5449) -> (-13.6937, -4.6265)
  line L6 (-13.6937, -4.6265) -> (225.987, -4.6265)
  line L7 (225.987, -4.6265) -> (225.987, 91.5449)
  line L8 (-10.6937, 88.5449) -> (222.987, 88.5449)
  line L9 (222.987, 88.5449) -> (222.987, -1.6265)
  line L10 (222.987, -1.6265) -> (-10.6937, -1.6265)
  line L11 (-10.6937, -1.6265) -> (-10.6937, 88.5449)
  constraint horizontal L8
  constraint vertical L9
  constraint horizontal L10
  constraint vertical L11
  constraint coincident L1.end L2.start
  constraint coincident L0.start L3.end
extrude "拉伸7" add sketch "草图4" along normal blind 1.5 separate body contours L0 L1 L2 L3 makes body 3
extrude "拉伸8" cut sketch "草图3" along normal blind 20 bodies 3
extrude "拉伸9" add 1 faces at (67.1999, -90.5449, 0) along direction (0, 0, 1) blind 1.5 on bodies 1 bodies 2 1 3
sketch "草图10" plane through (0, 4.6265, 0) normal (0, 1, 0) x (-1, 0, 0)
  line L0 (-190.9874, -1.5675) -> (-180.9874, -1.5675)
  line L1 (-180.9874, -1.5675) -> (-180.9874, -4.5675)
  line L2 (-180.9874, -4.5675) -> (-190.9874, -4.5675)
  line L3 (-190.9874, -4.5675) -> (-190.9874, -1.5675)
  line L4 (-225.987, 1.5) -> (-225.987, -8.5)
  line L5 (-225.987, -8.5) -> (13.6937, -8.5)
  line L6 (13.6937, -8.5) -> (13.6937, 1.5)
  line L7 (13.6937, 1.5) -> (-225.987, 1.5)
  line L8 (13.6937, -8.5) -> (-225.987, -8.5)
  line L9 (-225.987, -8.5) -> (-225.987, -11)
  line L10 (-225.987, -11) -> (13.6937, -11)
  line L11 (13.6937, -11) -> (13.6937, -8.5)
  dimension "d34" = 10
  dimension "d35" = 3
  constraint horizontal L0
  constraint vertical L1
  constraint horizontal L2
  constraint vertical L3
  measures "d34" distance of L0.start L0.end
  measures "d35" distance of L0.start L2.end
extrude "拉伸10" cut sketch "草图10" against normal blind 20 contours L0 L1 L2 L3 bodies 1 2
sketch "草图13" plane through (0, 0, -8.5) normal (0, 0, 1) x (-1, 0, 0)
  line L0 (-222.987, -1.6265) -> (10.6937, -1.6265)
  line L1 (10.6937, -1.6265) -> (10.6937, 88.5449)
  line L2 (10.6937, 88.5449) -> (-222.987, 88.5449)
  line L3 (-222.987, 88.5449) -> (-222.987, -1.6265)
  circle A0 centre (8.825, 0.2469) radius 0.2
  circle A1 centre (8.8437, 86.6812) radius 0.2
  circle A2 centre (-221.125, 0.25) radius 0.2
  circle A3 centre (-221.125, 86.6875) radius 0.2
  circle A4 centre (-49, 48) radius 0.2
  circle A5 centre (-163, 47.5) radius 0.2
  circle A6 centre (-106, 48) radius 0.2
  dimension "d47" = 0.4
  dimension "d48" = 0.4
  dimension "d49" = 0.4
  dimension "d50" = 0.4
  dimension "d51" = 0.4
  dimension "d52" = 0.4
  dimension "d53" = 0.4
  measures "d47" diameter of A0
  measures "d48" diameter of A1
  measures "d49" diameter of A2
  measures "d50" diameter of A3
  measures "d51" diameter of A4
  measures "d52" diameter of A5
  measures "d53" diameter of A6
extrude "拉伸11" add sketch "草图13" along normal blind 5.9 separate body contours A0 | A1 | A2 | A3 | A4 | A5 | A6 makes body 4 at (-9.0032, -86.802, -4.5667) makes body 5 at (105.804, -47.9604, -4.5667) makes body 6 at (221.12, -86.8874, -4.5667) makes body 7 at (-8.83, -0.4468, -4.5667) makes body 8 at (162.995, -47.6999, -4.5667) makes body 9 at (221.12, -0.4499, -4.5667) makes body 10 at (49.1396, -48.1432, -4.5667)
sketch "草图14" plane through (0, 0, -11) normal (0, 0, -1) x (1, 0, 0)
  line L0 (-10.6937, 88.5449) -> (222.987, 88.5449)
  line L1 (222.987, 88.5449) -> (222.987, -1.6265)
  line L2 (222.987, -1.6265) -> (-10.6937, -1.6265)
  line L3 (-10.6937, -1.6265) -> (-10.6937, 88.5449)
  line L4 (225.987, 91.5449) -> (-13.6937, 91.5449)
  line L5 (-13.6937, 91.5449) -> (-13.6937, -4.6265)
  line L6 (-13.6937, -4.6265) -> (225.987, -4.6265)
  line L7 (225.987, -4.6265) -> (225.987, 91.5449)
  circle A0 centre (-12, -3) radius 1.25
  circle A1 centre (-12, 90) radius 1.25
  circle A2 centre (224.5, 90) radius 1.25
  circle A3 centre (224.5, -3) radius 1.25
  dimension "d57" = 2.5
  dimension "d58" = 2.5
  dimension "d59" = 2.5
  dimension "d60" = 2.5
  measures "d57" diameter of A0
  measures "d58" diameter of A1
  measures "d59" diameter of A2
  measures "d60" diameter of A3
extrude "拉伸13" cut 1 faces at (67.1999, -90.5449, -11) along direction (0, 0, 1) blind 2.5 on bodies 2 bodies 2
sketch "草图15" plane through (0, 0, 0) normal (0, 0, 1) x (1, 0, 0)
sketch "草图16" plane through (0, 0, -8.5) normal (0, 0, -1) x (1, 0, 0)
  line L0 (-10.6937, 88.5449) -> (222.987, 88.5449)
  line L1 (222.987, 88.5449) -> (222.987, -1.6265)
  line L2 (222.987, -1.6265) -> (-10.6937, -1.6265)
  line L3 (-10.6937, -1.6265) -> (-10.6937, 88.5449)
  line L4 (225.987, 91.5449) -> (-13.6937, 91.5449)
  line L5 (-13.6937, 91.5449) -> (-13.6937, -4.6265)
  line L6 (-13.6937, -4.6265) -> (225.987, -4.6265)
  line L7 (225.987, -4.6265) -> (225.987, 91.5449)
  circle A0 centre (-12, -3) radius 1.25
  circle A1 centre (-12, 90) radius 1.25
  circle A2 centre (224.5, 90) radius 1.25
  circle A3 centre (224.5, -3) radius 1.25
  dimension "d65" = 2.5
  dimension "d66" = 2.5
  dimension "d67" = 2.5
  dimension "d68" = 2.5
  measures "d65" diameter of A0
  measures "d66" diameter of A1
  measures "d67" diameter of A2
  measures "d68" diameter of A3
extrude "拉伸14" cut sketch "草图16" against normal blind 5 contours A0 | A1 | A2 | A3 bodies 1
extrude "拉伸15" add 4 faces at (224.8443, -90.3589, -3.5) (224.1946, 2.7166, -3.5) (-12.2367, 2.5211, -3.5) (-11.6557, -90.3589, -3.5) along direction (0, 0, -1) blind 1.6 on bodies 1 bodies 1 2
fillet "圆角5" radius 2 1 edges at (106.1467, 4.6265, 1.5) on bodies 1
fillet "圆角6" radius 1.5 3 edges at (-13.6937, 4.6265, -4.5) (-13.6937, 4.0407, 0.9142) (-13.6937, -44.4592, 1.5) on bodies 1
fillet "圆角7" radius 1.5 3 edges at (-13.6937, -91.5449, -4.25) (-13.2543, -91.5449, 1.0607) (106.8967, -91.5449, 1.5) on bodies 1
fillet "圆角8" radius 1.5 5 edges at (225.987, -91.5449, -4.25) (225.987, -91.1055, 1.0607) (225.987, -43.7092, 1.5) (225.987, 4.0407, 0.9142) (225.987, 4.6265, -4.5) on bodies 1
extrude "拉伸12" [rolled back] along distance -2.5 taper angle 0
move_body "移动1" [rolled back] rotate angle 20
extrude "拉伸5" [rolled back] along distance -1.2 taper angle 0
